Autodesk Inventor part; units mm, degrees
(part 3 of 3)
  arc A242 (-142.5922, 103.3581) -> (-142.6462, 103.098) centre (-140.6652, 102.8226) ccw projected
  arc A243 (-141.6604, 103.9986) -> (-142.6462, 103.098) centre (-140.8817, 102.1564) ccw projected
  line L60 (-128.936, 109.3772) -> (-141.6604, 103.9986) projected
  arc A244 (-126.1727, 107.7823) -> (-128.936, 109.3772) centre (-128.1573, 107.535) ccw projected
  arc A245 (-132.0722, 89.6254) -> (-126.1727, 107.7823) centre (-148.5, 105) ccw projected
  arc A246 (-135.2453, 89.9594) -> (-132.0722, 89.6254) centre (-133.5325, 90.992) ccw projected
  line L61 (-142.378, 101.7899) -> (-135.2453, 89.9594) projected
  arc A247 (-142.6462, 103.098) -> (-142.378, 101.7899) centre (-140.6652, 102.8226) ccw projected
  line L62 (-166.9004, 112.9582) -> (-153.4448, 109.8304) projected
  arc A248 (-168.1986, 115.8727) -> (-166.9004, 112.9582) centre (-166.4476, 114.9063) ccw projected
  arc A249 (-152.7534, 127.0943) -> (-168.1986, 115.8727) centre (-148.5, 105) ccw projected
  arc A250 (-150.3827, 124.9591) -> (-152.7534, 127.0943) centre (-152.3753, 125.1304) ccw projected
  line L63 (-151.566, 111.1954) -> (-150.3827, 124.9591) projected
  arc A251 (-152.1179, 109.9796) -> (-151.566, 111.1954) centre (-153.5586, 111.3667) ccw projected
  arc A252 (-153.4448, 109.8304) -> (-152.1179, 109.9796) centre (-152.9919, 111.7784) ccw projected
  arc A253 (-145.434, 111.1954) -> (-144.8821, 109.9796) centre (-143.4414, 111.3667) ccw projected
  line L64 (-146.6173, 124.9591) -> (-145.434, 111.1954) projected
  arc A254 (-144.2466, 127.0943) -> (-146.6173, 124.9591) centre (-144.6247, 125.1304) ccw projected
  arc A255 (-128.8014, 115.8727) -> (-144.2466, 127.0943) centre (-148.5, 105) ccw projected
  arc A256 (-130.0996, 112.9582) -> (-128.8014, 115.8727) centre (-130.5524, 114.9063) ccw projected
  line L65 (-143.5552, 109.8304) -> (-130.0996, 112.9582) projected
  arc A257 (-144.8821, 109.9796) -> (-143.5552, 109.8304) centre (-144.0081, 111.7784) ccw projected
  point P0 (0, 0)
